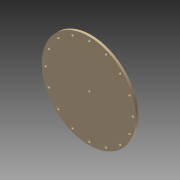
# Autodesk Inventor part: GE-13036
Saved by Autodesk Inventor 2013 (Build 170138000, 138)
## iProperties
Created: 2013-01-06
Part Number: GE-13036
Material: Polyethylene, High Density
Document SubType Name: Modeling
Designer: Phillip
Density: 1 g/cm^3
Author: Phillip
Autodesk Inventor part; units mm, degrees
ref_plane "YZ Plane" through (0, 0, 0) normal (1, 0, 0) x (0, 1, 0)
ref_plane "XZ Plane" through (0, 0, 0) normal (0, 1, 0) x (-1, 0, 0)
ref_plane "XY Plane" through (0, 0, 0) normal (0, 0, 1) x (1, 0, 0)
sketch "Sketch1" plane through (0, 0, 0) normal (0, 0, 1) x (1, 0, 0)
  circle A0 centre (0, 0) radius 127
  dimension "d2" = 254
  constraints: 1 centre point, 1 coincident
  measures "d2" diameter of A0
extrude "Extrusion1" add sketch "Sketch1" against normal blind 6.35
sketch "Sketch2" plane through (0, 0, 0) normal (0, 0, 1) x (1, 0, 0)
  circle A0 centre (0, 0) radius 127 projected
  constraints: 1 coincident
hole "Hole1" at (0, 0, 0) direction (0, 0, -1) diameter 6.858 end through all
sketch "Sketch3" plane through (0, 0, 0) normal (0, 0, 1) x (1, 0, 0)
  circle A0 centre (0, 0) radius 3.429 projected
  circle A1 centre (0, 0) radius 127 projected
  circle A2 centre (0, 0) radius 117.475 construction
  point P0 (0, 117.475)
  dimension "d11" = 234.95
  constraints: 2 vertical alignment, 1 coincident, 2 other
hole "Hole2" at (0, 117.475, 0) direction (0, 0, -1) diameter 7.874 end through all
pattern_circular "Circular Pattern1" count 16 over 360 about axis through (0, 0, 0) along (0, 0, -1) of "Hole2"
body "Solid1"
